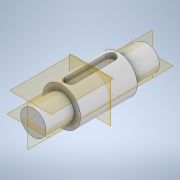
# Autodesk Inventor part: shaft1
Saved by Autodesk Inventor 2022 (Build 260153000, 153)
## iProperties
Created: 2023-12-21
Part Number: shaft1
Material: 一般
Document SubType Name: Modeling
Designer: ktamu
Density: 1 g/cm^3
Appearance: 既定
Author: ktamu
Autodesk Inventor part; units mm, degrees
sketch "スケッチ1" plane through (0, 0, 0) normal (0, 0, 1) x (1, 0, 0)
  circle A0 centre (0, 0) radius 15
  dimension "d0" = 30
  constraints: 1 centre point, 1 coincident
  measures "d0" diameter of A0
extrude "押し出し1" add sketch "スケッチ1" along normal blind 22.5
sketch "スケッチ2" plane through (0, 0, 22.5) normal (0, 0, 1) x (1, 0, 0)
  circle A0 centre (0, 0) radius 10
  dimension "d3" = 20
  constraints: 1 centre point, 1 coincident
  measures "d3" diameter of A0
extrude "押し出し2" add sketch "スケッチ2" along normal blind 22.5
ref_plane "作業平面1" through (0, 15, 0) normal (0, 1, 0) x (-1, 0, 0)
sketch "スケッチ3" plane through (0, 15, 0) normal (0, 1, 0) x (-1, 0, 0)
  line L0 (0, 0) -> (0, 20)
  line L1 (0, 20) -> (0, 16)
  arc A0 (4, 16) -> (0, 20) centre (0, 16) ccw
  arc A1 (0, 20) -> (-4, 16) centre (0, 16) ccw
  line L2 (4, 16) -> (4, 0)
  line L3 (-4, 16) -> (-4, 0)
  line L4 (4, 0) -> (-4, 0)
  dimension "d7" = 20
  dimension "d8" = 4
  constraints: 10 end point, 5 point on circle, 3 vertical, 2 centre point, 2 coincident, 1 concentric, 1 perpendicular, 1 point on line
  measures "d7" distance of L0.start L0.end
  measures "d8" distance of L0.end L1.end
extrude "押し出し3" cut sketch "スケッチ3" against normal blind 4
mirror "ミラー1" about plane through (0, 0, 0) normal (0, 0, 1) of "押し出し1", "押し出し2", "押し出し3"
